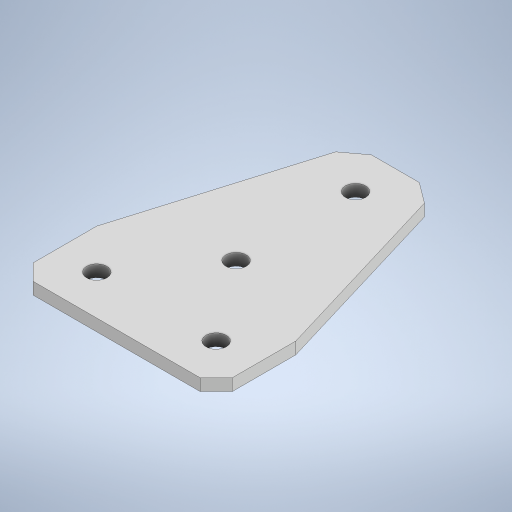
# Autodesk Inventor part: body_fix2
Saved by Autodesk Inventor 2024 (Build 280153000, 153)
## iProperties
Created: 2023-08-14
Part Number: body_fix2
Material: 常规
Document SubType Name: Modeling
Designer: wya
Density: 1 g/cm^3
Appearance: 默认
Author: wya
Autodesk Inventor part; units mm, degrees
ref_plane "YZ Plane" through (0, 0, 0) normal (1, 0, 0) x (0, 1, 0)
ref_plane "XZ Plane" through (0, 0, 0) normal (0, 1, 0) x (-1, 0, 0)
ref_plane "XY Plane" through (0, 0, 0) normal (0, 0, 1) x (1, 0, 0)
sketch "草图1" plane through (0, 0, 0) normal (0, 1, 0) x (-1, 0, 0)
  line L0 (0, 0) -> (50, 0)
  line L1 (50, 0) -> (50, -20)
  line L2 (50, -20) -> (0, -20)
  line L3 (0, -20) -> (0, 0)
  line L4 (35, -20) -> (15, -20)
  line L5 (15, -20) -> (15, -70)
  line L6 (15, -70) -> (35, -70)
  line L7 (35, -70) -> (35, -20)
  line L8 (25, 0) -> (25, -7.1636)
  line L9 (50, -20) -> (35, -70)
  line L10 (15, -70) -> (0, -20)
  circle A0 centre (40, -10) radius 2.55
  circle A1 centre (10, -10) radius 2.55
  circle A2 centre (25, -30) radius 2.55
  circle A3 centre (25, -60) radius 2.55
  line L11 (50, -10) -> (45.4992, -10)
  dimension "d0" = 50
  dimension "d1" = 20
  dimension "d2" = 20
  dimension "d3" = 50
  dimension "d4" = 5.1
  dimension "d5" = 10
  dimension "d6" = 10
  dimension "d7" = 10
  constraints: 24 end point, 5 point on line, 4 centre point, 4 parallel, 3 equal radius, 3 horizontal, 2 midpoint, 2 perpendicular, 1 symmetric about line, 1 vertical, 1 other
  measures "d0" distance between parallel lines of L3 L1
  measures "d1" distance between parallel lines of L2 L0
  measures "d2" distance of L5.end L6.end
  measures "d3" distance between parallel lines of L6 L2
  measures "d4" diameter of A0
  measures "d5" distance from line of A0.centre L1
  measures "d6" distance from line of L2 A2.centre
  measures "d7" distance from line of L6 A3.centre
extrude "拉伸1" add sketch "草图1" along normal blind 3
chamfer "倒角1" distance 4 angle 45 2 edges at (0, 1.5, 0) (-50, 1.5, 0)
chamfer "倒角2" distance 4 angle 45 2 edges at (-15, 1.5, -70) (-35, 1.5, -70)
